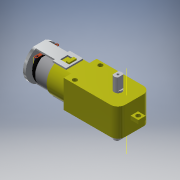
# Autodesk Inventor part: motor
Saved by Autodesk Inventor 2019 (Build 230136000, 136)
## iProperties
Created: 2017-01-12
Part Number: motor
Material: Generic
Document SubType Name: Modeling
Designer: schuer.davy
Density: 1 g/cm^3
Appearance: Default
Mass: 24.1387 g
Surface Area: 75.098 cm^2
Volume: 24.1387 cm^3
Author: schuer.davy
Autodesk Inventor part; units mm, degrees
sketch "Sketch1" plane through (0, 0, 0) normal (0, 0, 1) x (1, 0, 0)
  line L0 (6, -11.125) -> (-25.5, -11.125)
  line L1 (-25.5, -11.125) -> (-25.5, 11.125)
  line L2 (-25.5, 11.125) -> (6, 11.125)
  line L3 (11, 6.125) -> (11, -6.125)
  arc A0 (11, 6.125) -> (6, 11.125) centre (6, 6.125) ccw
  arc A1 (6, -11.125) -> (11, -6.125) centre (6, -6.125) ccw
  point P0 (0, 0)
  point P1 (11, -11.125)
  point P2 (11, 11.125)
  point P3 (11, 0)
  dimension "d0" = 36.5
  dimension "d1" = 11
  dimension "d2" = 22.25
  dimension "d3" = 5
  constraints: 8 end point, 4 point on circle, 4 point on line, 4 tangent, 2 centre point, 2 parallel, 1 equal radius, 1 horizontal, 1 horizontal alignment, 1 midpoint, 1 perpendicular
  measures "d0" distance of L1.end point (11, 11.125)
  measures "d1" distance from line of L3 point (0, 0)
  measures "d2" distance of point (11, 11.125) point (11, -11.125)
  measures "d3" radius of A0
extrude "Extrusion1" add sketch "Sketch1" along normal mid plane 18.75
sketch "Sketch2" plane through (0, 0, 9.375) normal (0, 0, 1) x (1, 0, 0)
  line L0 (-20.5, 8.6) -> (-20.5, -8.6) construction
  line L1 (-25.5, 11.125) -> (-25.5, -11.125) construction
  point P0 (0, 0)
  point P1 (-20.5, 0)
  dimension "d6" = 17.2
  dimension "d7" = 5
  constraints: 2 end point, 1 horizontal alignment, 1 midpoint, 1 vertical, 1 vertical alignment
  measures "d6" distance of L0.end L0.start
  measures "d7" distance between parallel lines of L1 L0
hole "Hole1" at (-20.5, 8.6, 9.375) at (-20.5, -8.6, 9.375) direction (0, 0, -1) diameter 3 end through all
ref_plane "Work Plane1" through (0, 0, 0) normal (0, 0, 1) x (1, 0, 0)
sketch "Sketch4" plane through (0, 0, 0) normal (0, 0, 1) x (1, 0, 0)
  line L0 (11, 6.125) -> (11, -6.125) projected
  line L1 (11, 2.5) -> (16.2, 2.5)
  line L2 (16.2, 2.5) -> (16.2, -2.5)
  line L3 (16.2, -2.5) -> (11, -2.5)
  line L4 (11, -2.5) -> (11, 2.5)
  circle A0 centre (13.6, 0) radius 1.5
  point P0 (0, 0)
  point P1 (16.2, 0)
  point P2 (13.6, 2.5)
  dimension "d16" = 5.2
  dimension "d17" = 5
  dimension "d18" = 3
  constraints: 8 end point, 2 horizontal alignment, 2 midpoint, 2 parallel, 1 centre point, 1 horizontal, 1 perpendicular, 1 point on line, 1 vertical alignment
  measures "d16" distance of L2.end L3.end
  measures "d17" distance of L1.end L2.end
  measures "d18" diameter of A0
extrude "Extrusion2" add sketch "Sketch4" along normal mid plane 2.5
sketch "Sketch5" plane through (-25.5, -11.125, 9.375) normal (-1, 0, 0) x (0, 0, 1)
  line L0 (0, 22.25) -> (-18.75, 22.25) projected
  line L1 (-18.75, 0) -> (-18.75, 22.25) projected
  line L2 (-18.75, 17.1146) -> (-18.75, 5.1354)
  line L3 (0, 22.25) -> (0, 0) projected
  line L4 (0, 17.1146) -> (0, 5.1354)
  arc A0 (-18.75, 5.1354) -> (0, 5.1354) centre (-9.375, 11.125) ccw
  arc A1 (0, 17.1146) -> (-18.75, 17.1146) centre (-9.375, 11.125) ccw
  line L5 (-18.75, 0) -> (0, 0) projected
  constraints: 4 end point, 4 point on circle, 4 point on line, 2 centre point, 2 tangent, 1 coincident
extrude "Extrusion3" add sketch "Sketch5" along normal blind 11.5 contours A1 L3 A0 L1
sketch "Sketch6" plane through (-37, -11.125, 9.375) normal (-1, 0, 0) x (0, 0, 1)
  line L0 (-18.75, 17.1146) -> (-18.75, 5.1354) projected
  arc A0 (-18.75, 5.1354) -> (0, 5.1354) centre (-9.375, 11.125) ccw projected
  line L1 (0, 5.1354) -> (0, 17.1146) projected
  arc A1 (0, 17.1146) -> (-18.75, 17.1146) centre (-9.375, 11.125) ccw projected
  line L2 (-17.55, 16.7531) -> (-17.55, 5.4969)
  arc A2 (-17.55, 5.4969) -> (-1.2, 5.4969) centre (-9.375, 11.125) ccw
  line L3 (-1.2, 5.4969) -> (-1.2, 16.7531)
  arc A3 (-1.2, 16.7531) -> (-17.55, 16.7531) centre (-9.375, 11.125) ccw
  dimension "d23" = 1.2
  constraints: 4 end point, 4 point on circle, 2 centre point, 3 other
  measures "d23" radial gap between concentric circles of A1 A3
extrude "Extrusion4" add sketch "Sketch6" along normal blind 14 contours A3 L3 A2 L2
sketch "Sketch7" plane through (0, 0, 0) normal (0, 0, 1) x (1, 0, 0)
  line L0 (-51, 9.925) -> (-51, 5.6281) projected
  line L1 (-37, 9.925) -> (-51, 9.925) projected
  arc A0 (-46, 9.925) -> (-51, 4.925) centre (-46, 4.925) ccw
  line L2 (-46, 9.925) -> (-51, 9.925)
  line L3 (-51, 9.925) -> (-51, 4.925)
  line L4 (-51, 5.6281) -> (-51, -5.6281) projected
  line L5 (-65.6826, 0) -> (29.8471, 0) projected
  point P0 (0, 0)
  dimension "d26" = 10
  constraints: 4 end point, 3 tangent, 2 point on circle, 2 point on line, 1 centre point, 1 collinear
  measures "d26" diameter of A0
revolve "Revolution1" cut sketch "Sketch7" angle 360 about axis through (-10, 0, 0) along (1, 0, 0)
sketch "Sketch8" plane through (0, 0, 9.375) normal (0, 0, 1) x (1, 0, 0)
  line L0 (-32.5, 2.5) -> (-30.5, 2.5)
  line L1 (-30.5, 2.5) -> (-30.5, -2.5)
  line L2 (-30.5, -2.5) -> (-32.5, -2.5)
  line L3 (-32.5, -2.5) -> (-32.5, 2.5)
  line L4 (-37, -5.9896) -> (-37, 5.9896) projected
  point P0 (0, 0)
  point P1 (-30.5, 0)
  dimension "d28" = 4.5
  dimension "d29" = 6.5
  dimension "d30" = 5
  constraints: 8 end point, 2 parallel, 1 horizontal, 1 horizontal alignment, 1 midpoint, 1 perpendicular
  measures "d28" distance between parallel lines of L4 L3
  measures "d29" distance between parallel lines of L1 L4
  measures "d30" distance of L2.end L0.start
extrude "Extrusion5" add sketch "Sketch8" along normal blind 2
sketch "Sketch9" plane through (-32.5, -2.5, 9.375) normal (0, -1, 0) x (1, 0, 0)
  line L0 (2, 1) -> (1, 1)
  line L1 (1, 1) -> (1, 0)
  line L2 (7, 0) -> (-4.5, 0) projected
  line L3 (0, 2) -> (2, 2) projected
  line L4 (0, 0) -> (0, 2) projected
  line L5 (2, 0) -> (0, 0) projected
  line L6 (2, 0) -> (2, 2) projected
  point P0 (32.5, -9.375)
  dimension "d33" = 1
  constraints: 4 end point, 2 midpoint, 2 perpendicular, 1 horizontal, 1 point on line
  measures "d33" distance between parallel lines of L3 L0
extrude "Extrusion6" cut sketch "Sketch9" against normal through all contours L6 L2 L1 L0
sketch "Sketch10" plane through (0, 0, -9.375) normal (0, 0, -1) x (-1, 0, 0)
  line L0 (32.5, -2.5) -> (32.5, 2.5) projected
  line L1 (32.5, -2.5) -> (30.5, -2.5) projected
  line L2 (30.5, 2.5) -> (32.5, 2.5) projected
  line L3 (30.5, -2.5) -> (30.5, 2.5) projected
  point P0 (0, 0)
extrude "Extrusion7" add sketch "Sketch10" along normal blind 2
sketch "Sketch11" plane through (-32.5, 2.5, -9.375) normal (0, 1, 0) x (1, 0, 0)
  line L0 (1, -19.75) -> (1, -18.75) projected
  line L1 (2, -19.75) -> (1, -19.75) projected
  line L2 (7, 0) -> (-4.5, 0) projected
  line L3 (2, 0) -> (2, 2) projected
  line L4 (0, 2) -> (2, 2) projected
  line L5 (7, 0) -> (-4.5, 0) projected
  line L6 (1, 0) -> (1, 1)
  line L7 (1, 1) -> (2, 1)
  point P0 (32.5, -9.375)
  constraints: 4 end point, 3 midpoint, 2 perpendicular, 1 horizontal, 1 point on line
extrude "Extrusion8" cut sketch "Sketch11" against normal through all
ref_plane "Work Plane2" through (-37, -5.6281, 8.075) normal (0, 0, 1) x (1, 0, 0)
sketch "Sketch16" plane through (-37, -5.6281, 8.075) normal (0, 0, 1) x (1, 0, 0)
  line L0 (0, 0) -> (-9, 0) projected
  line L1 (-9, 0) -> (-9, -4.2969) projected
  line L2 (-9, -1.8719) -> (-13.5, -1.8719)
  line L3 (-13.5, -1.8719) -> (-13.5, 13.1281)
  line L4 (-13.5, 13.1281) -> (-9, 13.1281)
  line L5 (-9, 13.1281) -> (-9, -1.8719)
  point P0 (37, 5.6281)
  point P1 (-13.5, 5.6281)
  dimension "d59" = 4.5
  dimension "d60" = 15
  constraints: 8 end point, 2 parallel, 1 horizontal, 1 horizontal alignment, 1 midpoint, 1 perpendicular, 1 point on line
  measures "d59" distance of L2.start L2.end
  measures "d60" distance of L2.end L3.end
extrude "Extrusion13" cut sketch "Sketch16" along normal blind 0.2
ref_plane "Work Plane3" through (-37, -5.6281, -8.075) normal (0, 0, -1) x (-1, 0, 0)
sketch "Sketch17" plane through (-37, -5.6281, -8.075) normal (0, 0, -1) x (-1, 0, 0)
  line L0 (13.5, 13.1281) -> (9, 13.1281) projected
  line L1 (13.5, -1.8719) -> (13.5, 13.1281) projected
  line L2 (9, 13.1281) -> (9, -1.8719) projected
  line L3 (9, -1.8719) -> (13.5, -1.8719) projected
  line L4 (9, 11.2561) -> (9, 0) projected
  point P0 (-37, 5.6281)
extrude "Extrusion14" cut sketch "Sketch17" along normal blind 0.2
sketch "Sketch18" plane through (-37, -5.6281, 8.075) normal (0, 0, 1) x (1, 0, 0)
  line L0 (-10.2, 13.1281) -> (-10.2, -1.8719)
  line L1 (-10.7, -2.3719) -> (-11.7, -2.3719)
  line L2 (53.2, 3.1281) -> (53.2, 8.1281) projected
  line L3 (-9, 11.2561) -> (-9, 0) projected
  line L4 (-10.7, 13.6281) -> (-11.7, 13.6281)
  line L5 (-12.2, 13.1281) -> (-12.2, -1.8719)
  line L6 (-12.2, 13.1281) -> (-11.7, 13.6281)
  line L7 (-10.7, 13.6281) -> (-10.2, 13.1281)
  line L8 (-10.2, -1.8719) -> (-10.7, -2.3719)
  line L9 (-11.7, -2.3719) -> (-12.2, -1.8719)
  line L10 (-11.2, 11.6281) -> (-11.2, 12.6281) construction
  line L11 (-10.7, 11.6281) -> (-10.7, 12.6281)
  line L12 (-11.7, 12.6281) -> (-11.7, 11.6281)
  arc A0 (-11.7, 11.6281) -> (-10.7, 11.6281) centre (-11.2, 11.6281) ccw
  arc A1 (-10.7, 12.6281) -> (-11.7, 12.6281) centre (-11.2, 12.6281) ccw
  line L13 (-27.44, 5.6281) -> (66.64, 5.6281) projected
  line L14 (-11.2, -0.3719) -> (-11.2, -1.3719) construction
  line L15 (-10.7, -0.3719) -> (-10.7, -1.3719)
  line L16 (-11.7, -1.3719) -> (-11.7, -0.3719)
  arc A2 (-10.7, -0.3719) -> (-11.7, -0.3719) centre (-11.2, -0.3719) ccw
  arc A3 (-11.7, -1.3719) -> (-10.7, -1.3719) centre (-11.2, -1.3719) ccw
  point P0 (37, 5.6281)
  point P1 (-10.2, -2.3719)
  point P2 (-10.2, 13.6281)
  point P3 (-12.2, -2.3719)
  point P4 (53.2, 5.6281)
  point P5 (-12.2, 13.6281)
  point P6 (-12.2, 5.6281)
  point P7 (-9, 5.6281)
  point P8 (-11.2, 12.1281)
  point P9 (-11.2, 13.6281)
  point P10 (-11.2, -0.8719)
  dimension "d66" = 1.2
  dimension "d67" = 16
  dimension "d68" = 2
  dimension "d69" = 0.5
  dimension "d70" = 0.5
  dimension "d71" = 0.5
  dimension "d72" = 0.5
  dimension "d73" = 0.5
  dimension "d74" = 0.5
  dimension "d75" = 0.5
  dimension "d76" = 0.5
  dimension "d77" = 0.5
  dimension "d78" = 1
  dimension "d79" = 1.5
  constraints: 32 end point, 8 point on circle, 8 point on line, 7 symmetric about line, 5 midpoint, 4 centre point, 4 parallel, 4 tangent, 1 horizontal, 1 horizontal alignment, 1 vertical alignment, 2 other
  measures "d66" distance between parallel lines of L0 L3
  measures "d67" distance of point (-12.2, 13.628) point (-12.2, -2.372)
  measures "d68" distance of point (-10.2, -2.372) point (-12.2, -2.372)
  measures "d69" distance of L5.start point (-12.2, 13.628)
  measures "d70" distance of L4.end point (-12.2, 13.628)
  measures "d71" distance of L4.start point (-10.2, 13.628)
  measures "d72" distance of L0.start point (-10.2, 13.628)
  measures "d73" distance of L0.end point (-10.2, -2.372)
  measures "d74" distance of L1.start point (-10.2, -2.372)
  measures "d75" distance of L1.end point (-12.2, -2.372)
  measures "d76" distance of L5.end point (-12.2, -2.372)
  measures "d77" radius of A1
  measures "d78" distance of L10.start L10.end
  measures "d79" distance from line of L4 point (-11.2, 12.128)
extrude "Extrusion15" add sketch "Sketch18" along normal blind 0.2
sketch "Sketch19" plane through (0, 0, 9.375) normal (0, 0, 1) x (1, 0, 0)
  circle A0 centre (0, 0) radius 2.6
  dimension "d82" = 5.2
  constraints: 1 centre point, 1 coincident
  measures "d82" diameter of A0
extrude "Extrusion16" add sketch "Sketch19" along normal blind 1.2
sketch "Sketch20" plane through (0, 0, 10.575) normal (0, 0, 1) x (1, 0, 0)
  circle A0 centre (0, 0) radius 2.6 projected
  line L0 (1.825, -1.8519) -> (1.825, 1.8519)
  circle A1 centre (0, 0) radius 2.6 projected
  line L1 (-1.825, -1.8519) -> (-1.825, 1.8519)
  circle A2 centre (0, 0) radius 0.75
  dimension "d85" = 3.65
  dimension "d86" = 1.5
  constraints: 7 point on circle, 4 end point, 2 vertical, 1 centre point, 1 coincident, 1 parallel
  measures "d85" distance between parallel lines of L1 L0
  measures "d86" diameter of A2
extrude "Extrusion17" add sketch "Sketch20" along normal blind 8 contours L0 A0 L1
sketch "Sketch21" plane through (0, 0, -9.375) normal (0, 0, -1) x (-1, 0, 0)
  circle A0 centre (0, 0) radius 2.6 projected
extrude "Extrusion18" add sketch "Sketch21" along normal blind 1.2
sketch "Sketch22" plane through (0, 0, -10.575) normal (0, 0, -1) x (-1, 0, 0)
  circle A0 centre (0, 0) radius 0.75 projected
  line L0 (-1.825, -1.8519) -> (-1.825, 1.8519) projected
  arc A1 (1.825, 1.8519) -> (-1.825, 1.8519) centre (0, 0) ccw projected
  line L1 (1.825, 1.8519) -> (1.825, -1.8519) projected
  arc A2 (-1.825, -1.8519) -> (1.825, -1.8519) centre (0, 0) ccw projected
extrude "Extrusion19" add sketch "Sketch22" along normal blind 8
sketch "Sketch23" plane through (-37, -5.6281, 8.075) normal (0, 0, 1) x (1, 0, 0)
  line L0 (-12.2, 2.2145) -> (-12.2, 9.0416) projected
  spline S0 degree 8 poles (-12.2, 2.2145) (-12.2168, 2.2505) (-12.2334, 2.2866) (-12.2496, 2.3229) (-12.2656, 2.3593) (-12.2814, 2.3958) (-12.2968, 2.4324) (-12.312, 2.4692) (-12.4772, 2.8775) (-12.6002, 3.2598) (-12.6985, 3.6499) (-12.7744, 4.0453) (-12.8298, 4.444) (-12.866, 4.8444) (-12.8837, 5.2457) (-12.8824, 5.9249) (-12.873, 6.2024) (-12.8548, 6.4796) (-12.8275, 6.7562) (-12.791, 7.0316) (-12.7446, 7.3055) (-12.6878, 7.5772) (-12.5907, 7.9618) (-12.5595, 8.077) (-12.5261, 8.1916) (-12.4906, 8.3056) (-12.4528, 8.4188) (-12.4128, 8.5312) (-12.3704, 8.6427) (-12.3108, 8.7897) (-12.2958, 8.826) (-12.2805, 8.8623) (-12.265, 8.8984) (-12.2491, 8.9344) (-12.233, 8.9703) (-12.2166, 9.006) (-12.2, 9.0416) knots 0 0 0 0 0 0 0 0 0 0.045389 0.045389 0.045389 0.045389 0.045389 0.045389 0.045389 0.502819 0.502819 0.502819 0.502819 0.502819 0.502819 0.502819 0.818988 0.818988 0.818988 0.818988 0.818988 0.818988 0.818988 0.955097 0.955097 0.955097 0.955097 0.955097 0.955097 0.955097 1 1 1 1 1 1 1 1 1 projected
  point P0 (37, 5.6281)
  constraints: 2 vertical alignment
extrude "Extrusion20" add sketch "Sketch23" along normal blind 0.8
ref_plane "Work Plane4" through (0, 0, 0) normal (0, 1, 0) x (1, 0, 0)
sketch "Sketch26" plane through (0, 0, 0) normal (0, 1, 0) x (1, 0, 0)
  line L0 (-49.1279, -8.875) -> (-46.7805, -8.875)
  line L1 (-46.7805, -8.875) -> (-46.7805, -8.275)
  line L2 (-46.7805, -8.275) -> (-49.1279, -8.275)
  line L3 (-49.1279, -8.275) -> (-49.1279, -8.875)
  line L4 (-47.2, -8.075) -> (-47.2, -8.275) projected
  line L5 (-46.7805, -8.275) -> (-47.2, -8.275)
  line L6 (-47.2, -8.275) -> (-47.2, -8.075)
  line L7 (-47.2, -8.075) -> (-46.7805, -8.075)
  line L8 (-46.7805, -8.075) -> (-46.7805, -8.275)
  point P0 (0, 0)
  constraints: 16 end point, 4 parallel, 2 horizontal, 2 perpendicular
extrude "Extrusion22" add sketch "Sketch26" along normal mid plane 7
sketch "Sketch28" plane through (-51, 0, 0) normal (-1, 0, 0) x (0, 0, 1)
  circle A0 centre (0, 0) radius 4.925 projected
  line L0 (-3.575, -3.3875) -> (-3.575, 3.3875)
  dimension "d108" = 8.5
  constraints: 2 end point, 2 point on circle, 1 vertical
extrude "Extrusion23" add sketch "Sketch28" along normal blind 2 contours A0 L0 picked at (-0.0531, 1.2782)
sketch "Sketch29" plane through (-53, 0, 0) normal (-1, 0, 0) x (0, 0, 1)
  circle A0 centre (0, 0) radius 1
  dimension "d111" = 2
  constraints: 1 centre point, 1 coincident
  measures "d111" diameter of A0
extrude "Extrusion24" add sketch "Sketch29" along normal blind 1
sketch "Sketch27" plane through (0, 0, 9.375) normal (0, 0, 1) x (1, 0, 0)
  line L0 (-29.3, -5.75) -> (-29.3, 5.75)
  line L1 (-29.3, 5.75) -> (-38.3, 5.75)
  line L2 (-38.3, 5.75) -> (-38.3, 4.25)
  line L3 (-38.3, 4.25) -> (-53, 4.25)
  line L4 (-53, 4.25) -> (-53, -4.25)
  line L5 (-53, -4.25) -> (-38.3, -4.25)
  line L6 (-38.3, -4.25) -> (-38.3, -5.75)
  line L7 (-38.3, -5.75) -> (-29.3, -5.75)
  line L8 (-32.5, 2.5) -> (-31.5, 2.5) projected
  line L9 (-31.5, 2.5) -> (-36.5, 2.5)
  line L10 (-36.5, 2.5) -> (-36.5, -2.5)
  line L11 (-31.5, -2.5) -> (-32.5, -2.5) projected
  line L12 (-36.5, -2.5) -> (-31.5, -2.5)
  line L13 (-31.5, -2.5) -> (-31.5, 2.5)
  line L14 (-68.9347, 0) -> (30.3891, 0) projected
  line L15 (-53, 4.925) -> (-53, -4.925) projected
  line L16 (-30.5, -2.5) -> (-30.5, 2.5) projected
  line L17 (-32.5, 2.5) -> (-32.5, -2.5) projected
  point P0 (0, 0)
  point P1 (-53, 0)
  point P2 (-29.3, 0)
  point P3 (-36.5, 0)
  point P4 (-53, -3.3875)
  point P5 (-53, 3.3875)
  point P6 (-38.3, 5)
  point P7 (-38.3, -5)
  dimension "d114" = 11.5
  dimension "d115" = 8.5
  dimension "d116" = 9
  dimension "d117" = 1.2
  dimension "d118" = 4
  constraints: 24 end point, 8 perpendicular, 5 midpoint, 3 point on line, 2 horizontal, 2 vertical, 1 collinear, 1 vertical alignment
  measures "d114" distance of L0.start L0.end
  measures "d115" distance of L3.end L4.end
  measures "d116" distance of L0.end L1.end
  measures "d117" distance between parallel lines of L0 L16
  measures "d118" distance between parallel lines of L17 L10
extrude "Extrusion25" add sketch "Sketch27" along normal up to surface (1 mm away)
extrude "Extrusion26" cut sketch "Sketch27" along normal up to next contours L17 L12 L10 L14 | L14 L10 L9 L17
sketch "Sketch30" plane through (0, 0, -9.375) normal (0, 0, -1) x (-1, 0, 0)
  line L0 (29.3, -5.75) -> (38.3, -5.75) projected
  line L1 (29.3, 5.75) -> (29.3, -5.75) projected
  line L2 (38.3, 5.75) -> (29.3, 5.75) projected
  line L3 (38.3, 4.25) -> (38.3, 5.75) projected
  line L4 (53, 4.25) -> (38.3, 4.25) projected
  line L5 (53, -4.25) -> (53, 4.25) projected
  line L6 (38.3, -4.25) -> (53, -4.25) projected
  line L7 (38.3, -5.75) -> (38.3, -4.25) projected
  line L8 (32.5, -2.5) -> (36.5, -2.5) projected
  line L9 (36.5, -2.5) -> (36.5, 2.5) projected
  line L10 (36.5, 2.5) -> (32.5, 2.5) projected
  line L11 (30.5, 2.5) -> (32.5, 2.5) projected
  line L12 (30.5, -2.5) -> (30.5, 2.5) projected
  line L13 (32.5, -2.5) -> (30.5, -2.5) projected
  point P0 (0, 0)
extrude "Extrusion27" add sketch "Sketch30" along normal up to surface (1 mm away)
sketch "Sketch31" plane through (-53, 0, 0) normal (-1, 0, 0) x (0, 0, 1)
  arc A0 (-3.575, -3.3875) -> (-3.575, 3.3875) centre (0, 0) ccw projected
  line L0 (-3.575, 3.3875) -> (-3.575, -3.3875) projected
  circle A1 centre (0, 0) radius 1 projected
  line L1 (-10.375, 4.25) -> (-10.375, -4.25) projected
  line L2 (10.375, -4.25) -> (10.375, 4.25) projected
  arc A2 (-10.375, -4.25) -> (10.375, -4.25) centre (0, 0) ccw
  arc A3 (10.375, 4.25) -> (-10.375, 4.25) centre (0, 0) ccw
  constraints: 4 end point, 4 point on circle, 2 centre point, 1 coincident
ref_plane "Work Plane5" through (-51, 0, 0) normal (-1, 0, 0) x (0, 0, 1)
sketch "Sketch32" plane through (-51, 0, 0) normal (-1, 0, 0) x (0, 0, 1)
  arc A0 (-10.375, -4.25) -> (10.375, -4.25) centre (0, 0) ccw projected
  arc A1 (10.375, 4.25) -> (-10.375, 4.25) centre (0, 0) ccw projected
  line L0 (-10.375, 4.25) -> (-10.375, -4.25) projected
  line L1 (10.375, -4.25) -> (10.375, 4.25) projected
  arc A2 (-3.575, -3.3875) -> (-3.575, 3.3875) centre (0, 0) ccw projected
  line L2 (-3.575, 3.3875) -> (-3.575, -3.3875) projected
extrude "Extrusion29" add sketch "Sketch32" along normal blind 1.9
scale "Scale1" factors (0.9, 0.9, 0.9) then translate (-5.1, 0, 0) bodies 1
scale "Scale2" factors (0.9, 0.9, 0.9) then translate (-5.1, 0, 0) bodies 1
equation "\"d70\" = d69"
equation "\"d71\" = d69"
equation "\"d72\" = d71"
equation "\"d73\" = d69"
equation "\"d74\" = d73"
equation "\"d75\" = d69"
equation "\"d76\" = d75"
body "Solid1"
